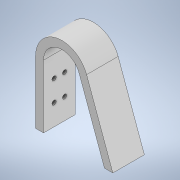
# Autodesk Inventor part: simpleLoopForLifting
Saved by Autodesk Inventor 2020.2 (Build 242310000, 310)
## iProperties
Created: 2020-01-11
Part Number: simpleLoopForLifting
Material: Generic
Document SubType Name: Modeling
Designer: robst
Density: 1 g/cm^3
Appearance: Default
Author: robst
Autodesk Inventor part; units mm, degrees
ref_plane "YZ Plane" through (0, 0, 0) normal (1, 0, 0) x (0, 1, 0)
ref_plane "XZ Plane" through (0, 0, 0) normal (0, 1, 0) x (-1, 0, 0)
ref_plane "XY Plane" through (0, 0, 0) normal (0, 0, 1) x (1, 0, 0)
sketch "Sketch1" plane through (0, 0, 0) normal (0, 0, 1) x (1, 0, 0)
  arc A0 (20.8847, 7.6014) -> (-22.225, 0) centre (0, 0) ccw
  line L0 (-22.225, 0) -> (-22.225, -76.2)
  line L1 (20.8847, 7.6014) -> (49.7358, -71.6664)
  line L2 (20.8847, 7.6014) -> (105.2397, 7.6014) construction
  arc A1 (30.8266, 7.6014) -> (-31.75, 0) centre (0, 0) ccw
  line L3 (-31.75, 0) -> (-31.75, -76.2)
  line L4 (-31.75, -76.2) -> (-22.225, -76.2)
  line L5 (59.8721, -71.6664) -> (29.8352, 10.8591)
  line L6 (-22.225, -76.2) -> (104.775, -76.2) construction
  line L7 (49.7358, -71.6664) -> (51.3859, -76.2)
  line L8 (59.8721, -71.6664) -> (61.5222, -76.2)
  line L9 (51.3859, -76.2) -> (61.5222, -76.2)
  dimension "d0" = 44.45
  dimension "d1" = 76.2
  dimension "d2" = 70
  dimension "d3" = 63.5
  dimension "d4" = 9.525
  dimension "d5" = 127
  constraints: 20 end point, 5 point on circle, 3 horizontal, 3 point on line, 3 tangent, 2 centre point, 2 coincident, 2 vertical, 1 collinear, 1 equal length, 1 parallel
  measures "d0" diameter of A0
  measures "d1" distance of L0.start L0.end
  measures "d2" angle of L1 L2
  measures "d3" diameter of A1
  measures "d4" distance between parallel lines of L5 L1
  measures "d5" distance of L0.end L6.end
extrude "Extrusion1" add sketch "Sketch1" along normal mid plane 38.1
sketch "Sketch2" plane through (-31.75, -76.2, 19.05) normal (-1, 0, 0) x (0, 0, 1)
  line L0 (-38.1, 0) -> (0, 0) construction
  line L1 (-12.7, 0) -> (-12.7, 76.2) construction
  line L2 (0, 76.2) -> (0, 0) projected
  line L3 (0, 0) -> (0, 76.2) construction
  line L4 (0, 25.4) -> (-38.1, 25.4) construction
  line L5 (-38.1, 76.2) -> (-38.1, 0) construction
  point P0 (-19.05, 76.2)
  point P1 (-12.7, 25.4)
  point P2 (-12.7, 50.8)
  point P3 (-25.4, 25.4)
  point P4 (-25.4, 50.8)
  dimension "d8" = 12.7
  dimension "d9" = 25.4
  dimension "d12" = 25.4
  dimension "d15" = 12.7
  constraints: 4 end point, 4 point on line, 2 horizontal, 2 vertical, 3 other
  measures "d8" distance between parallel lines of L2 L1
  measures "d9" distance from line of point (-12.7, 25.4) L0
  measures "d12" distance of point (-12.7, 25.4) point (-12.7, 50.8)
  measures "d15" distance of point (-12.7, 25.4) point (-25.4, 25.4)
hole "Hole1" at (-31.75, -50.8, 6.35) at (-31.75, -25.4, 6.35) at (-31.75, -50.8, -6.35) at (-31.75, -25.4, -6.35) direction (1, 0, 0) diameter 5.1054 depth 13.6144 tip angle 118 clearance for "Hex Machine Screw" size "#10" standard "Ansi Unified Screw Threads"
body "Solid1"
